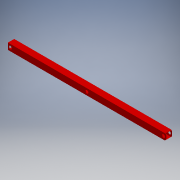
# Autodesk Inventor part: Long Bar Offset center
Saved by Autodesk Inventor 2018 (Build 220112000, 112)
## iProperties
Created: 2016-01-11
Part Number: Long Bar Offset center
Material: Generic
Document SubType Name: Modeling
Designer: Applegate
Density: 1 g/cm^3
Appearance: Default
Author: Applegate
Autodesk Inventor part; units mm, degrees
ref_plane "YZ Plane" through (0, 0, 0) normal (1, 0, 0) x (0, 1, 0)
ref_plane "XZ Plane" through (0, 0, 0) normal (0, 1, 0) x (-1, 0, 0)
ref_plane "XY Plane" through (0, 0, 0) normal (0, 0, 1) x (1, 0, 0)
sketch "Sketch1" plane through (0, 0, 0) normal (1, 0, 0) x (0, 1, 0)
  line L0 (-12.7, 12.7) -> (12.7, 12.7)
  line L1 (12.7, 12.7) -> (12.7, -12.7)
  line L2 (12.7, -12.7) -> (-12.7, -12.7)
  line L3 (-12.7, -12.7) -> (-12.7, 12.7)
  line L4 (-11.1125, 11.1125) -> (11.1125, 11.1125)
  line L5 (11.1125, 11.1125) -> (11.1125, -10.8514)
  line L6 (11.1125, -10.8514) -> (-11.1125, -10.8514)
  line L7 (-11.1125, -10.8514) -> (-11.1125, 11.1125)
  point P0 (0, 0)
  point P1 (0, 12.7)
  point P2 (-12.7, 0)
  dimension "d0" = 25.4
  dimension "d1" = 25.4
  dimension "d2" = 1.5875
  dimension "d3" = 1.5875
  dimension "d4" = 1.5875
  constraints: 16 end point, 4 parallel, 2 horizontal, 2 midpoint, 2 perpendicular, 1 horizontal alignment, 1 vertical alignment
  measures "d0" distance of L0.start L0.end
  measures "d1" distance of L2.end L0.start
  measures "d2" horizontal distance of L4.start L0.start
  measures "d3" horizontal distance of L2.end L6.end
  measures "d4" horizontal distance of L0.end L4.end
extrude "Extrusion1" add sketch "Sketch1" along normal blind 711.2
sketch "Sketch2" plane through (0, -12.7, 12.7) normal (0, 0, 1) x (1, 0, 0)
  circle A0 centre (9.525, 12.7) radius 6.35
  circle A1 centre (701.675, 12.7) radius 6.35
  line L0 (711.2, 25.4) -> (711.2, 0) projected
  line L1 (0, 0) -> (0, 25.4) projected
  line L2 (0, 0) -> (711.2, 0) projected
  circle A2 centre (355.6, 12.7) radius 6.35
  point P0 (0, 12.7)
  point P1 (395.7549, 0)
  point P2 (355.6, 0)
  dimension "d7" = 12.7
  dimension "d8" = 9.525
  dimension "d9" = 12.7
  dimension "d10" = 9.525
  dimension "d17" = 12.7
  dimension "d23" = 355.6
  dimension "BarLengthRef" = 711.2
  constraints: 3 centre point, 1 midpoint
  measures "d7" diameter of A0
  measures "d8" distance of A0.centre point (0, 12.7)
  measures "d9" diameter of A1
  measures "d10" distance from line of A1.centre L0
  measures "d17" diameter of A2
  measures "d23" distance from line of L1 A2.centre
  measures "BarLengthRef" distance from line of L0 point (0, 12.7)
extrude "Extrusion2" cut sketch "Sketch2" against normal blind 50.8 contours A0 | A1
extrude "Extrusion4" cut sketch "Sketch2" against normal blind 25.4 contours A2
fillet "Fillet1" radius 6.35 1 edges at (711.2, 12.7, 0)
fillet "Fillet2" radius 6.35 1 edges at (711.2, -12.7, 0)
equation "\"d1\" = d0"
equation "\"d3\" = d2"
equation "\"d4\" = d2"
equation "\"d9\" = d7"
equation "\"d10\" = d8"
equation "\"d17\" = d7"
equation "\"d23\" = 0.5 * BarLengthRef"
body "Solid1"
